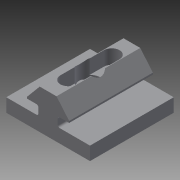
# Autodesk Inventor part: 2059_a
Saved by Autodesk Inventor 2014 SP2 (Build 180246200, 246)
## iProperties
Created: 2018-07-19
Part Number: 2059_a
Material: Generic
Catalog Web Link: www.cadenas.de
Description: 2059, 2051_a-Top Mount Bi-Fold Door Hanger Assembly
Vendor: 8020
Document SubType Name: Modeling
Designer: psadmin
Manufacturer: 8020
Mass: 3.62368 g
Surface Area: 26.6506 cm^2
Volume: 3.62368 cm^3
Density: 1 g/cm^3
Appearance: PSOLRGB-192-192-192
Category: PARTsolutions
Company: 8020
Title: 2059_a
Author: Cadenas PARTsolutions
Comments: Top Mount Bi-Fold Door Hanger Assembly
PSOL_IDENT_0: {$CADENAS_DATA\23d-libs\8020\inch\panels_and_doors\2059.prj},158 {VTYP=3D},{NB=2059_a},{LINA=2059_a}
PSOL_IDENT_1: ,{NN=2059, 2051_a},{DATE=16.03.2018 08:23:48},{GEOMDATE=24.01.2012 11:31:00},{VERSION=},{LINEID=10},
PSOL_IDENT_2: {WBVAR=},{WBNUMERIC=}  {NB=2059_a},{LINA=2059_a},{KT=DUMMY},{PN=2059},{DESC=Bi-Fold Door Hanger},{MA
PSOL_IDENT_3: T=UHMW Polyethylene},{L=1.000},{A=0.470},{B=1.000},{C=0.160},{D=0.110},{E=0.230},{F=0.200},{G=50},{T
PSOL_IDENT_4: S=1/4-20 x .410},{H=0.50207587},{R=0.025},{W=.045}
NN: 2059, 2051_a
NT: Top Mount Bi-Fold Door Hanger Assembly
NB: 2059_a
NBSYN: $PN._a
LINA: 2059_a
PN: 2059
DESC: Bi-Fold Door Hanger
MAT: UHMW Polyethylene
L: 1
A: 0.47
B: 1
C: 0.16
D: 0.11
E: 0.23
F: 0.2
G: 50
TS: 1/4-20 x .410
W: .045
SUPPLIER: 8020
ARTICLENO: 2059_a
BOMINFO: 2059_a
CREATOR: CADENAS GmbH
Autodesk Inventor part; units mm, degrees
sketch "Sketch_1" plane through (0, 0, 0) normal (0, 0, 1) x (1, 0, 0)
  line L0 (-12.7, 4.064) -> (-12.7, 0)
  line L1 (-12.7, 0) -> (12.7, 0)
  line L2 (12.7, 0) -> (12.7, 4.064)
  line L3 (12.7, 4.064) -> (3.556, 4.064)
  arc A0 (2.921, 4.699) -> (3.556, 4.064) centre (3.556, 4.699) ccw
  line L4 (2.921, 4.699) -> (2.921, 6.223)
  arc A1 (3.556, 6.858) -> (2.921, 6.223) centre (3.556, 6.223) ccw
  line L5 (3.556, 6.858) -> (6.3764, 6.858)
  line L6 (6.3764, 6.858) -> (6.3764, 7.366)
  line L7 (6.3764, 7.366) -> (2.54, 11.938)
  line L8 (2.54, 11.938) -> (-2.54, 11.938)
  line L9 (-2.54, 11.938) -> (-6.3764, 7.366)
  line L10 (-6.3764, 7.366) -> (-6.3764, 6.858)
  line L11 (-6.3764, 6.858) -> (-3.556, 6.858)
  arc A2 (-2.921, 6.223) -> (-3.556, 6.858) centre (-3.556, 6.223) ccw
  line L12 (-2.921, 6.223) -> (-2.921, 4.699)
  arc A3 (-3.556, 4.064) -> (-2.921, 4.699) centre (-3.556, 4.699) ccw
  line L13 (-3.556, 4.064) -> (-12.7, 4.064)
  constraints: 28 end point, 8 point on circle, 4 centre point
extrude "Extrusion1" add sketch "Sketch_1" along normal mid plane 25.4
sketch "Sketch_2" plane through (0, 11.938, 0) normal (0, 1, 0) x (1, 0, 0)
  line L0 (-2.3749, 6.604) -> (-2.3749, -6.604)
  arc A0 (-2.3749, -6.604) -> (2.3749, -6.604) centre (0, -6.604) ccw
  line L1 (2.3749, -6.604) -> (2.3749, 6.604)
  arc A1 (2.3749, 6.604) -> (-2.3749, 6.604) centre (0, 6.604) ccw
  constraints: 4 end point, 4 point on circle, 2 centre point
extrude "Extrusion2" cut sketch "Sketch_2" against normal blind 4.318
sketch "Sketch3" plane through (-12.7, 0, 12.7) normal (0, -1, 0) x (1, 0, 0)
  point P0 (12.7, -12.7)
hole "Hole1" at (0, 0, 0) direction (0, 1, 0) diameter 6.5278 depth 11.938
ref_plane "to_screw_XY" through (0, 0, 0) normal (0, -1, 0) x (1, 0, 0)
ref_plane "to_screw_YZ" through (0, 0, 0) normal (1, 0, 0) x (0, 0, 1)
ref_plane "to_screw_ZX" through (0, 0, 0) normal (0, 0, 1) x (0, -1, 0)
body "Solid1"
